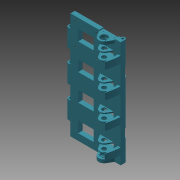
# Autodesk Inventor part: 砂轮架
Saved by Autodesk Inventor 2015 (Build 190159000, 159)
## iProperties
Created: 2017-05-16
Part Number: 砂轮架
Material: 常规
Document SubType Name: Modeling
Designer: Administrator
Density: 1 g/cm^3
Appearance: 灰蓝色
Author: Administrator
Autodesk Inventor part; units mm, degrees
ref_plane "YZ Plane" through (0, 0, 0) normal (1, 0, 0) x (0, 1, 0)
ref_plane "XZ Plane" through (0, 0, 0) normal (0, 1, 0) x (-1, 0, 0)
sketch "草图1" plane through (0, 0, 0) normal (0, 0, 1) x (1, 0, 0)
  line L0 (-227, 20) -> (0, 20)
  line L1 (0, 20) -> (0, 0)
  line L2 (0, 0) -> (-227, 0)
  line L3 (-227, 0) -> (-227, 5)
  arc A0 (-227, 20) -> (-227, 0) centre (-227, 10) ccw
  circle A1 centre (-227, 10) radius 5
  line L4 (0, 0) -> (-2, 0)
  line L5 (-2, 0) -> (-2, -60)
  line L6 (-2, -60) -> (0, -60)
  line L7 (0, -60) -> (0, 0)
  arc A2 (0, -60) -> (10.3373, 20) centre (-227, 10) ccw
  circle A3 centre (0.3462, 19.579) radius 10
  arc A4 (0, 9.585) -> (10.3373, 20) centre (0.3462, 19.579) ccw
  line L8 (0, 9.585) -> (0, -60)
  dimension "d2" = 10
  dimension "d0" = 227
  dimension "d1" = 20
  dimension "d3" = 2
  dimension "d4" = 60
  dimension "d5" = 20
  constraints: 18 end point, 8 point on circle, 4 centre point, 4 parallel, 4 tangent, 3 coincident, 2 horizontal, 2 perpendicular, 2 point on line, 1 collinear, 1 concentric, 1 vertical alignment, 2 other
  measures "d0" distance of L1.end L2.end
  measures "d1" distance of L0.end L1.end
  measures "d3" distance of L6.end L5.end
  measures "d4" distance of L4.end L5.end
  measures "d5" diameter of A3
extrude "拉伸1" add sketch "草图1" against normal blind 483
sketch "草图2" plane through (0, 0, -483) normal (0, 0, -1) x (-1, 0, 0)
  arc A0 (31.2154, -24.5) -> (72.7846, -24.5) centre (52, -12.5) ccw
  line L0 (17.0703, 0) -> (31.2154, -24.5)
  line L1 (72.7846, -24.5) -> (86.9297, 0)
  line L2 (2, 0) -> (227, 0) projected
  circle A1 centre (227, 10) radius 5 projected
  line L3 (17.0703, 0) -> (86.9297, 0)
  point P0 (0, 0)
  dimension "d8" = 48
  dimension "d9" = 120
  dimension "d10" = 175
  dimension "d11" = 22.5
  constraints: 6 end point, 2 point on circle, 2 point on line, 2 tangent, 1 centre point, 1 equal length
  measures "d8" diameter of A0
  measures "d9" angle of L2 L1
  measures "d10" horizontal distance of A1.centre A0.centre
  measures "d11" vertical distance of A1.centre A0.centre
extrude "拉伸2" add sketch "草图2" against normal blind 15 contours L0 L2 L1 A0
sketch "草图3" plane through (0, 0, -468) normal (0, 0, 1) x (1, 0, 0)
  circle A0 centre (-52, -12.5) radius 16
  arc A1 (-72.7846, -24.5) -> (-31.2154, -24.5) centre (-52, -12.5) ccw projected
  point P0 (0, 0)
  dimension "d14" = 32
  constraints: 1 centre point, 1 concentric
  measures "d14" diameter of A0
extrude "拉伸3" cut sketch "草图3" along normal mid plane 18
sketch "草图4" plane through (-52, -12.5, -477) normal (0, 0, 1) x (1, 0, 0)
  circle A0 centre (0, 0) radius 12
  arc A1 (-9.9875, 12.5) -> (9.9875, 12.5) centre (0, 0) ccw projected
  point P0 (52, 12.5)
  dimension "d17" = 24
  constraints: 1 centre point, 1 concentric
  measures "d17" diameter of A0
extrude "拉伸4" cut sketch "草图4" against normal blind 2
sketch "草图5" plane through (-52, -12.5, -479) normal (0, 0, 1) x (1, 0, 0)
  circle A0 centre (0, 0) radius 7.5
  circle A1 centre (0, 0) radius 12 projected
  point P0 (52, 12.5)
  dimension "d20" = 15
  constraints: 1 centre point, 1 concentric
  measures "d20" diameter of A0
extrude "拉伸5" cut sketch "草图5" against normal through all contours A0
sketch "草图6" plane through (-2, -60, 0) normal (-1, 0, 0) x (0, 0, 1)
  line L0 (0, 60) -> (-483, 60) projected
  line L1 (-483, 0) -> (-443, 0)
  line L2 (-443, 0) -> (-443, 60)
  line L3 (-443, 60) -> (-483, 60)
  line L4 (-483, 60) -> (-483, 0)
  line L5 (0, 0) -> (-483, 0) projected
  line L6 (-413, 0) -> (-323, 0)
  line L7 (-323, 0) -> (-323, 60)
  line L8 (-323, 60) -> (-413, 60)
  line L9 (-413, 60) -> (-413, 0)
  line L10 (-293, 0) -> (-203, 0)
  line L11 (-203, 0) -> (-203, 60)
  line L12 (-203, 60) -> (-293, 60)
  line L13 (-293, 60) -> (-293, 0)
  line L14 (-173, 0) -> (-83, 0)
  line L15 (-83, 0) -> (-83, 60)
  line L16 (-83, 60) -> (-173, 60)
  line L17 (-173, 60) -> (-173, 0)
  line L18 (0, 0) -> (-53, 0)
  line L19 (-53, 0) -> (-53, 60)
  line L20 (-53, 60) -> (0, 60)
  line L21 (0, 60) -> (0, 0)
  dimension "d23" = 40
  dimension "d24" = 90
  dimension "d25" = 30
  dimension "d26" = 90
  dimension "d27" = 30
  dimension "d28" = 30
  dimension "d29" = 90
  dimension "d78" = 53
  dimension "d79" = 30
  constraints: 40 end point, 10 parallel, 8 point on line, 5 horizontal, 5 perpendicular
  measures "d23" distance of L3.end L2.end
  measures "d24" distance of L8.end L7.end
  measures "d25" distance between parallel lines of L2 L9
  measures "d26" distance of L12.end L11.end
  measures "d27" distance between parallel lines of L7 L13
  measures "d28" distance between parallel lines of L11 L17
  measures "d29" distance of L15.end L16.end
  measures "d78" distance between parallel lines of L21 L19
  measures "d79" distance between parallel lines of L15 L19
extrude "拉伸6" cut sketch "草图6" against normal through all contours L21 L5 L19 L0 | L15 L5 L17 L0 | L11 L5 L13 L0 | L7 L5 L9 L0 | L2 L1 L4 L0
sketch "草图7" plane through (0, 0, -468) normal (0, 0, 1) x (1, 0, 0)
  arc A0 (-69.3205, -22.5) -> (-34.6795, -22.5) centre (-52, -12.5) ccw
  circle A1 centre (-52, -12.5) radius 7.5 projected
  line L0 (-34.6795, -22.5) -> (-21.6891, 0)
  line L1 (-227, 0) -> (10.3373, 0) projected
  line L2 (-69.3205, -22.5) -> (-82.3109, 0)
  line L3 (-21.6891, 0) -> (-82.3109, 0)
  line L4 (-31.2154, -24.5) -> (-17.0703, 0) projected
  line L5 (-86.9297, 0) -> (-72.7846, -24.5) projected
  circle A2 centre (-52, -12.5) radius 7.5 projected
  circle A3 centre (-52, -12.5) radius 12 projected
  point P0 (0, 0)
  dimension "d33" = 40
  constraints: 6 end point, 2 parallel, 2 point on circle, 2 point on line, 2 tangent, 1 centre point, 1 collinear, 1 concentric
  measures "d33" diameter of A0
extrude "拉伸7" add sketch "草图7" along normal blind 420 contours L2 L1 L0 A0 | A3
sketch "草图8" plane through (-227, 0, 0) normal (0, -1, 0) x (1, 0, 0)
  line L0 (205.3109, -48) -> (205.3109, -468) projected
  line L1 (144.6891, -468) -> (205.3109, -468)
  line L2 (205.3109, -468) -> (205.3109, -448)
  line L3 (205.3109, -448) -> (144.6891, -448)
  line L4 (144.6891, -448) -> (144.6891, -468)
  line L5 (144.6891, -468) -> (144.6891, -48) projected
  line L6 (144.6891, -443) -> (205.3109, -443)
  line L7 (205.3109, -443) -> (205.3109, -413)
  line L8 (205.3109, -413) -> (144.6891, -413)
  line L9 (144.6891, -413) -> (144.6891, -443)
  line L10 (205.3109, -408) -> (144.6891, -408)
  line L11 (144.6891, -408) -> (144.6891, -328)
  line L12 (144.6891, -328) -> (205.3109, -328)
  line L13 (205.3109, -328) -> (205.3109, -408)
  line L14 (144.6891, -323) -> (205.3109, -323)
  line L15 (205.3109, -323) -> (205.3109, -293)
  line L16 (205.3109, -293) -> (144.6891, -293)
  line L17 (144.6891, -293) -> (144.6891, -323)
  line L18 (205.3109, -288) -> (144.6891, -288)
  line L19 (144.6891, -288) -> (144.6891, -208)
  line L20 (144.6891, -208) -> (205.3109, -208)
  line L21 (205.3109, -208) -> (205.3109, -288)
  line L22 (205.3109, -203) -> (144.6891, -203)
  line L23 (144.6891, -203) -> (144.6891, -173)
  line L24 (144.6891, -173) -> (205.3109, -173)
  line L25 (205.3109, -173) -> (205.3109, -203)
  line L26 (205.3109, -168) -> (144.6891, -168)
  line L27 (144.6891, -168) -> (144.6891, -88)
  line L28 (144.6891, -88) -> (205.3109, -88)
  line L29 (205.3109, -88) -> (205.3109, -168)
  line L30 (205.3109, -83) -> (144.6891, -83)
  line L31 (144.6891, -83) -> (144.6891, -53)
  line L32 (144.6891, -53) -> (205.3109, -53)
  line L33 (205.3109, -53) -> (205.3109, -83)
  line L34 (192.3205, -48) -> (157.6795, -48) projected
  point P0 (227, 0)
  dimension "d37" = 20
  dimension "d38" = 5
  dimension "d39" = 30
  dimension "d40" = 5
  dimension "d41" = 80
  dimension "d42" = 5
  dimension "d43" = 30
  dimension "d44" = 5
  dimension "d45" = 80
  dimension "d46" = 5
  dimension "d47" = 30
  dimension "d48" = 5
  dimension "d49" = 80
  dimension "d50" = 5
  dimension "d51" = 30
  dimension "d52" = 5
  constraints: 64 end point, 16 parallel, 8 horizontal, 8 perpendicular, 17 other
  measures "d37" distance of L3.end L1.start
  measures "d38" distance between parallel lines of L3 L6
  measures "d39" distance between parallel lines of L6 L8
  measures "d40" distance between parallel lines of L8 L10
  measures "d41" distance of L10.end L11.end
  measures "d42" distance between parallel lines of L12 L14
  measures "d43" distance of L16.end L14.start
  measures "d44" distance between parallel lines of L16 L18
  measures "d45" distance of L18.end L19.end
  measures "d46" distance between parallel lines of L20 L22
  measures "d47" distance of L22.end L23.end
  measures "d48" distance between parallel lines of L24 L26
  measures "d49" distance between parallel lines of L28 L26
  measures "d50" distance between parallel lines of L28 L30
  measures "d51" distance between parallel lines of L30 L32
  measures "d52" distance between parallel lines of L34 L32
extrude "拉伸8" cut sketch "草图8" along normal through all contours L0 L30 L5 L32 | L0 L26 L5 L28 | L0 L22 L5 L24 | L0 L18 L5 L20 | L0 L14 L5 L16 | L0 L10 L5 L12 | L0 L6 L5 L8 | L0 L1 L4 L3
sketch "草图10" plane through (0, 0, -48) normal (0, 0, 1) x (1, 0, 0)
  circle A0 centre (-52, -12.5) radius 10
  circle A1 centre (-52, -12.5) radius 7.5 projected
  circle A2 centre (-52, -12.5) radius 7.5
  point P0 (0, 0)
  dimension "d55" = 20
  constraints: 2 centre point, 2 concentric, 1 coincident
  measures "d55" diameter of A0
extrude "拉伸9" cut sketch "草图10" against normal up to surface (400 mm away)
sketch "草图11" plane through (0, 0, -48) normal (0, 0, 1) x (1, 0, 0)
  circle A0 centre (-52, -12.5) radius 10
  circle A1 centre (-52, -12.5) radius 7.5 projected
  line L0 (-44.8397, -4.9019) -> (-41.8397, -10.0981)
  line L1 (-42.2386, -10.3284) -> (-40.4541, -9.2981)
  line L2 (-40.4541, -9.2981) -> (-43.4541, -4.1019)
  line L3 (-43.4541, -4.1019) -> (-45.2386, -5.1322)
  circle A2 centre (-52, -12.5) radius 10 projected
  line L4 (-31.2154, -24.5) -> (-17.0703, 0) projected
  point P0 (0, 0)
  point P1 (-43.3397, -7.5)
  dimension "d58" = 20
  dimension "d59" = 1.6
  dimension "d60" = 6
  dimension "d61" = 30
  constraints: 8 end point, 3 perpendicular, 3 point on circle, 2 point on line, 1 centre point, 1 concentric, 1 midpoint, 1 tangent
  measures "d58" diameter of A0
  measures "d59" distance between parallel lines of L0 L2
  measures "d60" distance between parallel lines of L1 L3
  measures "d61" angle of L4 L1
extrude "拉伸10" cut sketch "草图11" against normal blind 5 contours A0 L0 L1 | L3 L0 A0 | L0 L3 L2 L1
pattern_linear "矩形阵列1" count 4 spacing 120 along (0, 0, -1) of "拉伸10"
sketch "草图12" plane through (0, 0, 0) normal (0, 0, 1) x (1, 0, 0)
  arc A0 (-72.7846, -24.5) -> (-31.2154, -24.5) centre (-52, -12.5) ccw
  arc A1 (-72.7846, -24.5) -> (-31.2154, -24.5) centre (-52, -12.5) ccw projected
  line L0 (-72.7846, -24.5) -> (-86.9297, 0)
  arc A2 (-72.7846, -24.5) -> (-31.2154, -24.5) centre (-52, -12.5) ccw projected
  line L1 (-72.7846, -24.5) -> (-86.9297, 0) projected
  line L2 (-86.9297, 0) -> (-17.0703, 0)
  line L3 (-17.0703, 0) -> (-31.2154, -24.5)
  line L4 (-17.0703, 0) -> (-31.2154, -24.5) projected
  point P0 (0, 0)
  dimension "d67" = 48
  constraints: 6 end point, 4 tangent, 2 collinear, 2 point on circle, 2 point on line, 1 centre point, 1 horizontal
  measures "d67" diameter of A0
extrude "拉伸11" add sketch "草图12" against normal blind 18
sketch "草图13" plane through (0, 0, 0) normal (0, 0, 1) x (1, 0, 0)
  circle A0 centre (-52, -12.5) radius 16
  arc A1 (-72.7846, -24.5) -> (-31.2154, -24.5) centre (-52, -12.5) ccw projected
  point P0 (0, 0)
  dimension "d70" = 32
  constraints: 1 centre point, 1 concentric
  measures "d70" diameter of A0
extrude "拉伸12" cut sketch "草图13" against normal blind 18
sketch "草图14" plane through (-227, 0, -483) normal (0, -1, 0) x (1, 0, 0)
  line L0 (144.6891, 40) -> (205.3109, 40)
  line L1 (205.3109, 40) -> (205.3109, 70)
  line L2 (205.3109, 70) -> (144.6891, 70)
  line L3 (144.6891, 70) -> (144.6891, 40)
  point P0 (227, 483)
  constraints: 8 end point, 2 parallel, 1 horizontal, 1 perpendicular
extrude "拉伸13" cut sketch "草图14" against normal blind 20
pattern_linear "矩形阵列2" count 4 spacing 120 along (0, 0, 1) of "拉伸13"
sketch "草图15" plane through (0, 0, 0) normal (0, 0, 1) x (1, 0, 0)
  circle A0 centre (-52, -12.5) radius 24
  arc A1 (-72.7846, -24.5) -> (-31.2154, -24.5) centre (-52, -12.5) ccw projected
  line L0 (-31.2154, -24.5) -> (-17.0703, 0)
  line L1 (-31.2154, -24.5) -> (-17.0703, 0) projected
  line L2 (-17.0703, 0) -> (-17.0703, 20)
  line L3 (-17.0703, 20) -> (-86.9297, 20)
  line L4 (-227, 20) -> (-9.645, 20) projected
  line L5 (-86.9297, 0) -> (-86.9297, 20)
  line L6 (-86.9297, 0) -> (-72.7846, -24.5)
  line L7 (-86.9297, 0) -> (-72.7846, -24.5) projected
  line L8 (-9.645, 20) -> (-227, 20) projected
  point P0 (0, 0)
  dimension "d80" = 48
  constraints: 10 end point, 2 collinear, 2 perpendicular, 2 tangent, 1 centre point, 1 point on line, 1 vertical
  measures "d80" diameter of A0
extrude "拉伸14" cut sketch "草图15" against normal blind 5
sketch "草图16" plane through (0, 0, -5) normal (0, 0, 1) x (1, 0, 0)
  circle A0 centre (-27.0703, 10) radius 1.5
  circle A1 centre (-76.9297, 10) radius 1.5
  circle A2 centre (-69.3205, -22.5) radius 1.5
  circle A3 centre (-34.6795, -22.5) radius 1.5
  arc A4 (-69.3205, -22.5) -> (-34.6795, -22.5) centre (-52, -12.5) ccw
  arc A5 (-72.7846, -24.5) -> (-31.2154, -24.5) centre (-52, -12.5) ccw projected
  line L0 (-17.0703, 20) -> (-17.0703, 0) projected
  line L1 (-86.9297, 20) -> (-17.0703, 20) projected
  line L2 (-86.9297, 0) -> (-86.9297, 20) projected
  point P0 (0, 0)
  dimension "d83" = 3
  dimension "d84" = 3
  dimension "d85" = 3
  dimension "d86" = 3
  dimension "d87" = 20
  dimension "d88" = 10
  dimension "d89" = 10
  dimension "d90" = 10
  dimension "d91" = 10
  dimension "d92" = 10
  dimension "d93" = 10
  constraints: 5 centre point, 2 point on circle, 1 concentric
  measures "d83" diameter of A0
  measures "d84" diameter of A1
  measures "d85" diameter of A2
  measures "d86" diameter of A3
  measures "d87" radius of A4
  measures "d88" vertical distance of A2.centre A4.centre
  measures "d89" vertical distance of A4.centre A3.centre
  measures "d90" distance from line of L0 A0.centre
  measures "d91" distance from line of L1 A0.centre
  measures "d92" distance from line of L1 A1.centre
  measures "d93" distance from line of L2 A1.centre
extrude "拉伸15" cut sketch "草图16" against normal blind 13
thread "螺纹1" size "M3x0.5" class "6H" standard "ANSI Metric M Profile" full length
thread "螺纹2" size "M3x0.5" class "6H" standard "ANSI Metric M Profile" full length
thread "螺纹3" size "M3x0.5" class "6H" standard "ANSI Metric M Profile" full length
thread "螺纹4" size "M3x0.5" class "6H" standard "ANSI Metric M Profile" full length
sketch "草图17" plane through (-227, 20, -483) normal (0, 1, 0) x (1, 0, 0)
  line L0 (0, -483) -> (140.0703, -483) projected
  line L1 (-10, -483) -> (-10, 0) projected
  line L2 (10, -483) -> (-10, -483)
  line L3 (-10, -483) -> (-10, -423)
  line L4 (-10, -423) -> (10, -423)
  line L5 (10, -423) -> (10, -483)
  line L6 (-10, -342) -> (10, -342)
  line L7 (10, -342) -> (10, -282)
  line L8 (10, -282) -> (-10, -282)
  line L9 (-10, -282) -> (-10, -342)
  line L10 (-10, -201) -> (10, -201)
  line L11 (10, -201) -> (10, -141)
  line L12 (10, -141) -> (-10, -141)
  line L13 (-10, -141) -> (-10, -201)
  line L14 (-10, -60) -> (10, -60)
  line L15 (10, -60) -> (10, 0)
  line L16 (10, 0) -> (-10, 0)
  line L17 (-10, 0) -> (-10, -60)
  line L18 (0, 0) -> (217.355, 0) projected
  point P0 (227, -483)
  dimension "d104" = 60
  dimension "d105" = 20
  dimension "d106" = 81
  dimension "d107" = 81
  dimension "d108" = 81
  constraints: 32 end point, 8 parallel, 6 point on line, 5 collinear, 4 horizontal, 4 perpendicular
  measures "d104" distance of L14.end L15.end
  measures "d105" distance of L14.start L14.end
  measures "d106" distance between parallel lines of L12 L14
  measures "d107" distance between parallel lines of L8 L10
  measures "d108" distance between parallel lines of L4 L6
extrude "拉伸16" cut sketch "草图17" against normal through all
sketch "草图18" plane through (-9.645, 20, 0) normal (0, 1, 0) x (1, 0, 0)
  circle A0 centre (-184.855, 20) radius 4
  circle A1 centre (-89.855, 20) radius 4
  circle A2 centre (-184.855, 120) radius 4
  circle A3 centre (-89.855, 120) radius 4
  line L0 (-77.2847, 0) -> (-207.355, 0) projected
  line L1 (-217.355, 60) -> (-217.355, 141) projected
  point P0 (9.645, 0)
  dimension "d111" = 8
  dimension "d112" = 8
  dimension "d113" = 8
  dimension "d114" = 8
  dimension "d115" = 20
  dimension "d116" = 20
  dimension "d117" = 120
  dimension "d118" = 120
  dimension "d119" = 32.5
  dimension "d120" = 32.5
  dimension "d121" = 95
  dimension "d122" = 95
  constraints: 4 centre point
  measures "d111" diameter of A0
  measures "d112" diameter of A1
  measures "d113" diameter of A2
  measures "d114" diameter of A3
  measures "d115" distance from line of L0 A0.centre
  measures "d116" distance from line of L0 A1.centre
  measures "d117" distance from line of L0 A3.centre
  measures "d118" distance from line of L0 A2.centre
  measures "d119" distance from line of L1 A0.centre
  measures "d120" distance from line of L1 A2.centre
  measures "d121" distance of A3.centre A2.centre
  measures "d122" distance of A0.centre A1.centre
extrude "拉伸17" cut sketch "草图18" against normal blind 20
thread "螺纹5" size "M8x1.25" class "6H" standard "ANSI Metric M Profile" full length
thread "螺纹6" size "M8x1.25" class "6H" standard "ANSI Metric M Profile" full length
thread "螺纹7" size "M8x1.25" class "6H" standard "ANSI Metric M Profile" full length
thread "螺纹8" size "M8x1.25" class "6H" standard "ANSI Metric M Profile" full length
sketch "草图19" plane through (-9.645, 20, 0) normal (0, 1, 0) x (1, 0, 0)
  line L0 (-172.6659, 93) -> (-102.6659, 93)
  line L1 (-102.6659, 93) -> (-102.6659, 43)
  line L2 (-102.6659, 43) -> (-172.6659, 43)
  line L3 (-172.6659, 43) -> (-172.6659, 93)
  line L4 (-72.6659, 83) -> (-12.0442, 83) projected
  line L5 (-12.0442, 53) -> (-72.6659, 53) projected
  line L6 (-72.6659, 53) -> (-72.6659, 83) projected
  point P0 (9.645, 0)
  dimension "d133" = 70
  dimension "d134" = 10
  dimension "d135" = 10
  dimension "d136" = 30
  constraints: 8 end point, 2 parallel, 1 horizontal, 1 perpendicular
  measures "d133" distance of L0.start L0.end
  measures "d134" distance between parallel lines of L4 L0
  measures "d135" distance between parallel lines of L5 L2
  measures "d136" distance between parallel lines of L6 L1
extrude "拉伸18" cut sketch "草图19" against normal through all
pattern_linear "矩形阵列3" count 4 spacing 120 along (0, 0, -1) of "拉伸18"
sketch "草图20" plane through (0, 0, 0) normal (0, 0, 1) x (1, 0, 0)
  circle A0 centre (0.3462, 19.579) radius 5
  arc A1 (10.3373, 20) -> (-9.645, 20) centre (0.3462, 19.579) ccw projected
  point P0 (0, 0)
  dimension "d142" = 10
  constraints: 1 centre point, 1 concentric
  measures "d142" diameter of A0
extrude "拉伸19" cut sketch "草图20" against normal through all
ref_plane "工作平面1" through (0, 0, -108) normal (0, 0, 1) x (1, 0, 0)
sketch "草图21" plane through (0, 0, -108) normal (0, 0, 1) x (1, 0, 0)
  circle A0 centre (0.3462, 19.579) radius 10
  arc A1 (10.3373, 20) -> (-9.645, 20) centre (0.3462, 19.579) ccw projected
  point P0 (0, 0)
  dimension "d146" = 20
  constraints: 1 centre point, 1 concentric
  measures "d146" diameter of A0
extrude "拉伸20" cut sketch "草图21" against normal blind 40
pattern_linear "矩形阵列4" count 2 spacing 240 along (0, 0, -1) of "拉伸20"
